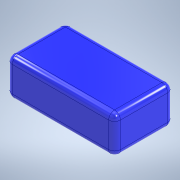
# Autodesk Inventor part: Bateria
Saved by Autodesk Inventor 2021 (Build 250183000, 183)
## iProperties
Created: 2022-03-22
Part Number: Bateria
Material: Generic
Document SubType Name: Modeling
Designer: Matheus
Density: 1.50085 g/cm^3
Appearance: Blue - Wall Paint - Glossy
Mass: 45.9 g
Surface Area: 59.8416 cm^2
Volume: 30.5827 cm^3
Author: Matheus
Autodesk Inventor part; units mm, degrees
ref_plane "YZ Plane" through (0, 0, 0) normal (1, 0, 0) x (0, 1, 0)
ref_plane "XZ Plane" through (0, 0, 0) normal (0, 1, 0) x (-1, 0, 0)
ref_plane "XY Plane" through (0, 0, 0) normal (0, 0, 1) x (1, 0, 0)
sketch "Sketch1" plane through (0, 0, 0) normal (0, 0, 1) x (1, 0, 0)
  line L0 (-27.5, -9.5) -> (27.5, -9.5)
  line L1 (27.5, -9.5) -> (27.5, 9.5)
  line L2 (27.5, 9.5) -> (-27.5, 9.5)
  line L3 (-27.5, 9.5) -> (-27.5, -9.5)
  line L4 (-27.5, -9.5) -> (27.5, 9.5) construction
  line L5 (27.5, -9.5) -> (-27.5, 9.5) construction
  point P0 (0, 0)
  dimension "d0" = 55
  dimension "d1" = 19
  constraints: 12 end point, 2 midpoint, 2 parallel, 1 horizontal, 1 perpendicular
  measures "d0" distance of L2.end L1.end
  measures "d1" distance of L1.end L0.end
extrude "Extrusion1" add sketch "Sketch1" against normal mid plane 30
fillet "Fillet1" radius 3 12 edges at (0, 9.5, 15) (-27.5, 9.5, 0) (0, 9.5, -15) (27.5, 9.5, 0) (27.5, 0, 15) (-27.5, 0, 15) (0, -9.5, 15) (27.5, -9.5, 0) (27.5, 0, -15) (-27.5, 0, -15) (0, -9.5, -15) (-27.5, -9.5, 0)
body "Solid1"
